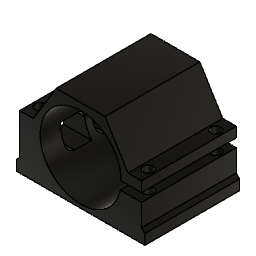
Frugy (Autodesk Fusion 360 archive; units mm, degrees)
design "BRACKET MOTOR JGA25-370 Rv Version"
Autodesk Fusion 360 part; units mm, degrees
sketch "Sketch1" plane through (0, 0, 0) normal (0, 1, 0) x (1, 0, 0)
  line L0 (-7.2239, -14.083) -> (-14, -3)
  line L1 (-18, -3) -> (-14, -3)
  line L2 (-18, -3) -> (-18, 0)
  line L3 (0, 4) -> (0, 6)
  line L4 (0, 12) -> (-19, 12)
  line L5 (-19, 12) -> (-19, 10)
  line L6 (-19, 10) -> (-18, 9)
  line L7 (-18, 9) -> (-18, 0)
  line L8 (7.2239, -14.083) -> (14, -3)
  line L9 (18, -3) -> (14, -3)
  line L10 (18, -3) -> (18, 0)
  line L11 (18, 9) -> (18, 2.5)
  line L12 (19, 10) -> (18, 9)
  line L13 (19, 12) -> (19, 10)
  line L14 (0, 12) -> (19, 12)
  line L15 (-7.2239, -14.083) -> (7.2239, -14.083)
  line L16 (12, 0) -> (18, 0)
  line L17 (11.7367, 2.5) -> (18, 2.5)
  arc A0 (11.7367, 2.5) -> (12, 0) centre (0, 0) ccw
  dimension "d1" = 24
  dimension "d6" = 4
  dimension "d8" = 2.5
  constraint coincident A0.centre origin
  constraint perpendicular L1 L2
  constraint vertical L3
  constraint coincident L4.start A0
  constraint horizontal L4
  constraint perpendicular L4 L5
  constraint symmetric L0.start L3 L8.start
  constraint symmetric L1.start L3 L9.start
  constraint symmetric L0.end L3 L8.end
  constraint symmetric L2.end L3 L10.end
  constraint symmetric L3 L4.start L14.start
  constraint symmetric L3 L4.end L13.start
  constraint symmetric L3 L5.end L12.start
  constraint symmetric L3 L6.end L11.start
  constraint perpendicular L10 L16
  constraint perpendicular L11 L17
  measures "d1" diameter of A0
  measures "d6" distance of L1.start L0.end
  measures "d8" distance of L16 L17
extrude "Extrude1" add sketch "Sketch1" along normal blind 30
sketch "Sketch3" plane through (0, 0, 3) normal (0, 0, 1) x (-1, 0, 0)
  line L0 (18, 0) -> (14, 0)
  line L1 (14, 0) -> (14, -30)
  line L2 (14, -30) -> (18, -30)
  line L3 (18, -30) -> (18, 0)
  circle A0 centre (16, -26) radius 1.5
  circle A1 centre (16, -6) radius 1.5
  line L4 (-18, 0) -> (-14, 0)
  line L5 (-14, -30) -> (-18, -30)
  circle A2 centre (-16, -6) radius 1.5
  line L6 (-14, 0) -> (-14, -30)
  circle A3 centre (-16, -26) radius 1.5
  dimension "d14" = 2
  dimension "d15" = 4
  dimension "d16" = 3
  dimension "d17" = 2
  dimension "d33" = 6
  dimension "d38" = 6
  dimension "d40" = 2
  dimension "d41" = 3
  dimension "d42" = 3
  dimension "d43" = 2
  dimension "d44" = 3
  dimension "d45" = 4
  dimension "d46" = 2
  measures "d14" distance of L1 A0.centre
  measures "d15" distance of L2 A0.centre
  measures "d16" diameter of A0
  measures "d17" distance of L3 A0.centre
  measures "d33" distance of L0 A1.centre
  measures "d38" distance of L4 A2.centre
  measures "d40" distance of A2.centre L6
  measures "d41" diameter of A1
  measures "d42" diameter of A2
  measures "d43" distance of L1 A1.centre
  measures "d44" diameter of A3
  measures "d45" distance of L5 A3.centre
  measures "d46" distance of L6 A3.centre
extrude "Extrude3" cut sketch "Sketch3" against normal blind 19 contours A0 | A1
sketch "Sketch4" plane through (-18, 0, 0) normal (-1, 0, 0) x (0, -1, 0)
  line L0 (0, -9) -> (0, 0)
  line L1 (0, 0) -> (-30, 0)
  line L2 (-30, 0) -> (-30, -9)
  line L3 (-30, -9) -> (0, -9)
  line L4 (-13, 0) -> (-8, 0)
  line L5 (-8, 0) -> (-8, -5)
  line L6 (-19, -7) -> (-24, -7)
  line L7 (-24, -7) -> (-24, -2)
  arc A0 (-22, 0) -> (-24, -2) centre (-22, -2) ccw
  arc A1 (-10, -7) -> (-8, -5) centre (-10, -5) ccw
  line L8 (-15, -2) -> (-15, -7)
  line L9 (-17, 0) -> (-17, -5)
  arc A2 (-19, -7) -> (-17, -5) centre (-19, -5) ccw
  line L10 (-15, -7) -> (-10, -7)
  arc A3 (-13, 0) -> (-15, -2) centre (-13, -2) ccw
  line L11 (-22, 0) -> (-17, 0)
  dimension "d20" = 2
  dimension "d23" = 6
  dimension "d24" = 8
  dimension "d27" = 2
  dimension "d28" = 2
  dimension "d47" = 2
  constraint horizontal L4
  constraint vertical L5
  constraint horizontal L6
  constraint vertical L7
  constraint tangent L4 A0
  constraint tangent L7 A0
  constraint tangent L6 A1
  constraint tangent L5 A1
  constraint equal A0 A1
  constraint coincident L6 A1.start
  constraint tangent L6 A2
  constraint tangent L9 A2
  constraint tangent A1 L10
  constraint coincident L4 A0.start
  constraint tangent L4 A3
  constraint tangent L8 A3
  measures "d20" radius of A0
  measures "d23" distance of L2 L7
  measures "d24" distance of L0 L5
  measures "d27" radius of A2
  measures "d28" radius of A3
  measures "d47" distance of L8 L9
extrude "Extrude5" cut sketch "Sketch4" against normal blind 10 contours L1 L4 L5 A1 L8 L10 A3 | L1 L6 L7 A0 L9 A2 L11
extrude "Extrude6" add 2 faces at (6.3333, 20, -12) (-4.9202, 12.2817, -12) along direction (0, 0, -1) blind 3
extrude "Extrude7" cut sketch "Sketch3" against normal blind 21 contours A2 | A3
extrude "Extrude8" cut 1 faces at (-15.86, 0, -4.0491) along direction (0, 1, 0) blind 2
sketch "Sketch6" plane through (0, 30, 0) normal (0, 1, 0) x (-1, 0, 0)
  arc A0 (-11.7367, -2.5) -> (-12, 0) centre (0, 0) ccw
  line L0 (-11.7367, -2.5) -> (-18, -2.5)
  line L1 (-18, -2.5) -> (-18, -9)
  line L2 (-18, -9) -> (-19, -10)
  line L3 (-19, -10) -> (-19, -15)
  line L4 (-19, -15) -> (19, -15)
  line L5 (19, -15) -> (19, -10)
  line L6 (19, -10) -> (18, -9)
  line L7 (18, -9) -> (18, 0)
  line L8 (18, 0) -> (18, 3)
  line L9 (18, 3) -> (14, 3)
  line L10 (14, 3) -> (7.2239, 14.083)
  line L11 (7.2239, 14.083) -> (-7.2239, 14.083)
  line L12 (-7.2239, 14.083) -> (-14, 3)
  line L13 (-14, 3) -> (-18, 3)
  line L14 (-18, 3) -> (-18, 0)
  line L15 (-18, 0) -> (-12, 0)
  line L16 (-19, -13) -> (19, -13)
  line L17 (0, -12) -> (0.2, -12)
  line L18 (-19, -15) -> (19, -15)
  line L19 (19, -13) -> (19, -15)
  line L20 (-19, -13) -> (-19, -15)
  dimension "d53" = 1
  dimension "d54" = 38
  dimension "d55" = 38
  dimension "d56" = 2
  constraint coincident L3 L16.start
  constraint coincident L5 L16.end
  constraint perpendicular L5 L16
  constraint coincident A0 L17.start
  constraint horizontal L17
  constraint coincident L3.end L4.start
  constraint coincident L4.end L5.start
  measures "d53" distance of L16 L17
  measures "d54" distance of L16.start L16.end
  measures "d55" distance of L3.end L4.end
  measures "d56" distance of L16.start L3.end
extrude "Extrude9" cut sketch "Sketch6" against normal blind 50 contours L3 L4 L5 L16 L18 L19 L20
named bodies: "BRACKET MOTOR"
